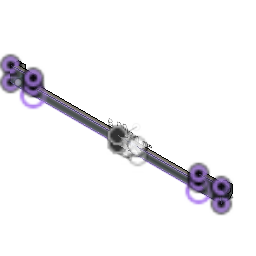
_NewBackstopA.91023b1a-daad-4caa-a02c-d6031eac0186 (Autodesk Fusion 360 design; units mm, degrees)
Autodesk Fusion 360 part; units mm, degrees
sketch "Sketch1" plane through (0, 0, 0) normal (0, 1, 0) x (1, 0, 0)
  line L0 (0, 0) -> (-25, 0)
  line L1 (-25, 0) -> (-25, -5)
  line L2 (-25, -5) -> (5, -5)
  line L3 (0, 0) -> (0, 10)
  line L4 (0, 10) -> (5, 10)
  line L5 (5, 10) -> (5, -5)
  line L6 (-25, 0) -> (-245, 0)
  line L7 (-245, 0) -> (-245, -5)
  line L8 (-245, -5) -> (-25, -5)
  line L9 (-25, 0) -> (-140, 0)
  line L10 (-140, 0) -> (-140, 27.0089)
  line L11 (-270, 10) -> (-275, 10)
  line L12 (-270, 0) -> (-270, 10)
  line L13 (-275, 10) -> (-275, -5)
  line L14 (-270, 0) -> (-245, 0)
  line L15 (-245, -5) -> (-275, -5)
  line L16 (-245, 0) -> (-245, -5)
  point P0 (-270, 0)
  dimension "d1" = 25
  dimension "d2" = 5
  dimension "d3" = 30
  dimension "d4" = 10
  dimension "d5" = 5
  dimension "d6" = 220
  dimension "d7" = 5
  dimension "d8" = 115
  constraint coincident L0.start L3.start
  constraint horizontal L0
  constraint perpendicular L0 L1
  constraint perpendicular L1 L2
  constraint perpendicular L0 L3
  constraint perpendicular L3 L4
  constraint perpendicular L1 L6
  constraint perpendicular L6 L7
  constraint perpendicular L1 L9
  constraint perpendicular L6 L10
  measures "d1" distance of L0.start L0.end
  measures "d2" distance of L0.end L1.end
  measures "d3" distance of L1.end L2.end
  measures "d4" distance of L0.start L3.end
  measures "d5" distance of L3.end L4.end
  measures "d6" distance of L0.end L6.end
  measures "d7" distance of L6.end L7.end
  measures "d8" distance of L0.end L9.end
extrude "Extrude1" add sketch "Sketch1" along normal blind 10
extrude "Extrude2" add sketch "Sketch1" along normal blind 20 contours L0 L1 L2 L3 L4 L5 | L7 L11 L12 L13 L14 L15 L16
sketch "Sketch2" plane through (5, 0, 0) normal (1, 0, 0) x (0, 0, -1)
  line L0 (-5, 0) -> (10, 0)
  line L1 (10, 0) -> (10, 20)
  line L2 (10, 20) -> (-5, 20)
  line L3 (-5, 20) -> (-5, 0)
sketch "Sketch3" plane through (0, 0, 0) normal (-1, 0, 0) x (0, 0, 1)
  line L0 (-10, 0) -> (0, 0)
  line L1 (0, 0) -> (0, 20)
  line L2 (0, 20) -> (-10, 20)
  line L3 (-10, 20) -> (-10, 0)
  line L4 (-10, 0) -> (-5, 0)
  line L5 (-5, 0) -> (-5, 10)
  circle A0 centre (-5, 10) radius 2.5
  dimension "d13" = 5
  dimension "d14" = 10
  dimension "d15" = 5
  constraint coincident L0.start L3.end
  constraint midpoint L0 L4.end
  constraint perpendicular L4 L5
  constraint coincident L5.end A0.centre
  measures "d13" distance of L0.start L4.end
  measures "d14" distance of L4.end L5.end
  measures "d15" diameter of A0
extrude "Extrude3" cut sketch "Sketch3" along normal mid plane 662 contours A0
chamfer "Chamfer1" distance 5 angle 45 4 edges at (2.5, 20, -10) (2.5, 0, -10) (-272.5, 20, -10) (-272.5, 0, -10)
sketch "Sketch4" plane through (0, 0, 5) normal (0, 0, 1) x (1, 0, 0)
  line L0 (-25, 10) -> (-245, 10)
  line L1 (-245, 10) -> (-245, 20)
  line L2 (-245, 20) -> (-275, 20)
  line L3 (-275, 20) -> (-275, 0)
  line L4 (-275, 0) -> (5, 0)
  line L5 (5, 0) -> (5, 20)
  line L6 (5, 20) -> (-25, 20)
  line L7 (-25, 20) -> (-25, 10)
  line L8 (-127.0455, 8) -> (-132.9543, 6.9581)
  line L9 (-127.0455, 8) -> (-127.0455, 2)
  line L10 (-127.0455, 8) -> (-121.0455, 8) construction
  line L11 (-132.9543, 0) -> (-106, 0)
  line L12 (-132.9543, 3.0419) -> (-132.9543, 0)
  line L13 (-132.9543, 6.9581) -> (-132.9543, 10)
  line L14 (-132.9543, 10) -> (-107.3817, 10)
  line L15 (-127.0455, 2) -> (-132.9543, 3.0419)
  line L16 (-127.0455, 2) -> (-121.0455, 2) construction
  line L17 (-245, 0) -> (-25, 0)
  point P0 (-130, 10)
  dimension "d19" = 6
  dimension "d20" = 170
  dimension "d21" = 6
  dimension "d22" = 170
  dimension "d23" = 6
  constraint vertical L9
  constraint horizontal L10
  constraint horizontal L16
  constraint vertical L13
  constraint coincident L0 L13.end
  constraint coincident L11.start L17
  constraint coincident L9.end L15.start
  measures "d19" distance of L8.start L9.end
  measures "d20" angle of L8 L10
  measures "d21" distance of L8.end L8.start
  measures "d22" angle of L15 L16
  measures "d23" distance of L9.end L12.start
extrude "Extrude4" [rolled back] along distance -30 taper angle 0
